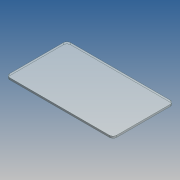
# Autodesk Inventor part: P019_EcranProtecLidar
Saved by Autodesk Inventor 2021.3 (Build 253353000, 353)
## iProperties
Created: 2021-11-12
Part Number: P019_EcranProtecLidar
Material: Glass
Document SubType Name: Modeling
Designer: gabri
Density: 2.18 g/cm^3
Appearance: Clear
Author: gabri
Autodesk Inventor part; units mm, degrees
ref_plane "YZ Plane" through (0, 0, 0) normal (1, 0, 0) x (0, 1, 0)
ref_plane "XZ Plane" through (0, 0, 0) normal (0, 1, 0) x (-1, 0, 0)
ref_plane "XY Plane" through (0, 0, 0) normal (0, 0, 1) x (1, 0, 0)
sketch "Sketch2" plane through (0, 0, 0) normal (0, 0, 1) x (1, 0, 0)
  line L0 (29, -16.5) -> (-29, -16.5)
  line L1 (-29, -16.5) -> (-29, 16.5)
  line L2 (-29, 16.5) -> (29, 16.5)
  line L3 (29, 16.5) -> (29, -16.5)
  line L4 (29, -16.5) -> (-29, 16.5) construction
  line L5 (-29, -16.5) -> (29, 16.5) construction
  point P0 (0, 0)
  dimension "d0" = 58
  dimension "d1" = 33
  constraints: 12 end point, 2 midpoint, 2 parallel, 1 horizontal, 1 perpendicular
  measures "d0" distance of L1.end L2.end
  measures "d1" distance of L0.end L1.end
extrude "Extrusion1" add sketch "Sketch2" along normal blind 1
fillet "Fillet1" radius 2 4 edges at (-29, -16.5, 0.5) (29, -16.5, 0.5) (29, 16.5, 0.5) (-29, 16.5, 0.5)
body "Solid1"
